Autodesk Inventor part; units mm, degrees
(part 3 of 3)
sketch "Sketch8" plane through (390.9, -150.3, 0) normal (0, 0, 1) x (0, 1, 0)
  line L0 (44.94, -15.18) -> (44.94, 14.82) projected
  line L1 (44.94, 14.82) -> (54.94, 14.82) projected
  line L2 (54.94, 14.82) -> (54.94, -15.18) projected
  line L3 (54.94, -15.18) -> (44.94, -15.18) projected
  line L4 (-55.06, -15.18) -> (-55.06, 14.82) projected
  line L5 (-55.06, 14.82) -> (-45.06, 14.82) projected
  line L6 (-45.06, 14.82) -> (-45.06, -15.18) projected
  line L7 (-45.06, -15.18) -> (-55.06, -15.18) projected
  circle A0 centre (56.765, -50.18) radius 1.7 projected
  circle A1 centre (56.765, 49.82) radius 1.7 projected
  circle A2 centre (-56.885, -50.18) radius 1.7 projected
  circle A3 centre (-56.885, 49.82) radius 1.7 projected
  line L8 (56.765, 74.82) -> (56.765, 86.645) projected
  line L9 (56.765, 86.645) -> (54.94, 86.645) projected
  line L10 (54.94, 86.645) -> (54.94, 89.82) projected
  line L11 (54.94, 89.82) -> (44.94, 89.82) projected
  line L12 (44.94, 89.82) -> (44.94, 86.645) projected
  line L13 (44.94, 86.645) -> (34.94, 86.645) projected
  line L14 (34.94, 86.645) -> (34.94, 89.82) projected
  line L15 (34.94, 89.82) -> (24.94, 89.82) projected
  line L16 (24.94, 89.82) -> (24.94, 86.645) projected
  line L17 (24.94, 86.645) -> (14.94, 86.645) projected
  line L18 (14.94, 86.645) -> (14.94, 89.82) projected
  line L19 (14.94, 89.82) -> (4.94, 89.82) projected
  line L20 (4.94, 89.82) -> (4.94, 86.645) projected
  line L21 (4.94, 86.645) -> (-5.06, 86.645) projected
  line L22 (-5.06, 86.645) -> (-5.06, 89.82) projected
  line L23 (-5.06, 89.82) -> (-15.06, 89.82) projected
  line L24 (-15.06, 89.82) -> (-15.06, 86.645) projected
  line L25 (-15.06, 86.645) -> (-25.06, 86.645) projected
  line L26 (-25.06, 86.645) -> (-25.06, 89.82) projected
  line L27 (-25.06, 89.82) -> (-35.06, 89.82) projected
  line L28 (-35.06, 89.82) -> (-35.06, 86.645) projected
  line L29 (-35.06, 86.645) -> (-45.06, 86.645) projected
  line L30 (-45.06, 86.645) -> (-45.06, 89.82) projected
  line L31 (-45.06, 89.82) -> (-55.06, 89.82) projected
  line L32 (-55.06, 89.82) -> (-55.06, 86.645) projected
  line L33 (-55.06, 86.645) -> (-56.885, 86.645) projected
  line L34 (-56.885, 86.645) -> (-56.885, 74.82) projected
  line L35 (-56.885, 74.82) -> (-60.06, 74.82) projected
  line L36 (-60.06, 74.82) -> (-60.06, 64.82) projected
  line L37 (-60.06, 64.82) -> (-56.885, 64.82) projected
  line L38 (-56.885, 64.82) -> (-56.885, 54.82) projected
  line L39 (-56.885, 54.82) -> (-60.06, 54.82) projected
  line L40 (-60.06, 54.82) -> (-60.06, 44.82) projected
  line L41 (-60.06, 44.82) -> (-56.885, 44.82) projected
  line L42 (-56.885, 44.82) -> (-56.885, 34.82) projected
  line L43 (-56.885, 34.82) -> (-60.06, 34.82) projected
  line L44 (-60.06, 34.82) -> (-60.06, 24.82) projected
  line L45 (-60.06, 24.82) -> (-56.885, 24.82) projected
  line L46 (-56.885, 24.82) -> (-56.885, 14.82) projected
  line L47 (-56.885, 14.82) -> (-60.06, 14.82) projected
  line L48 (-60.06, 14.82) -> (-60.06, 4.82) projected
  line L49 (-60.06, 4.82) -> (-56.885, 4.82) projected
  line L50 (-56.885, 4.82) -> (-56.885, -5.18) projected
  line L51 (-56.885, -5.18) -> (-60.06, -5.18) projected
  line L52 (-60.06, -5.18) -> (-60.06, -15.18) projected
  line L53 (-60.06, -15.18) -> (-56.885, -15.18) projected
  line L54 (-56.885, -15.18) -> (-56.885, -25.18) projected
  line L55 (-56.885, -25.18) -> (-60.06, -25.18) projected
  line L56 (-60.06, -25.18) -> (-60.06, -35.18) projected
  line L57 (-60.06, -35.18) -> (-56.885, -35.18) projected
  line L58 (-56.885, -35.18) -> (-56.885, -45.18) projected
  line L59 (-56.885, -45.18) -> (-60.06, -45.18) projected
  line L60 (-60.06, -45.18) -> (-60.06, -55.18) projected
  line L61 (-60.06, -55.18) -> (-56.885, -55.18) projected
  line L62 (-56.885, -55.18) -> (-56.885, -65.18) projected
  line L63 (-56.885, -65.18) -> (-60.06, -65.18) projected
  line L64 (-60.06, -65.18) -> (-60.06, -75.18) projected
  line L65 (-60.06, -75.18) -> (-56.885, -75.18) projected
  line L66 (-56.885, -75.18) -> (-56.885, -87.005) projected
  line L67 (-56.885, -87.005) -> (-55.06, -87.005) projected
  line L68 (-55.06, -87.005) -> (-55.06, -90.18) projected
  line L69 (-55.06, -90.18) -> (-45.06, -90.18) projected
  line L70 (-45.06, -90.18) -> (-45.06, -87.005) projected
  line L71 (-45.06, -87.005) -> (-35.06, -87.005) projected
  line L72 (-35.06, -87.005) -> (-35.06, -90.18) projected
  line L73 (-35.06, -90.18) -> (-25.06, -90.18) projected
  line L74 (-25.06, -90.18) -> (-25.06, -87.005) projected
  line L75 (-25.06, -87.005) -> (-15.06, -87.005) projected
  line L76 (-15.06, -87.005) -> (-15.06, -90.18) projected
  line L77 (-15.06, -90.18) -> (-5.06, -90.18) projected
  line L78 (-5.06, -90.18) -> (-5.06, -87.005) projected
  line L79 (-5.06, -87.005) -> (4.94, -87.005) projected
  line L80 (4.94, -87.005) -> (4.94, -90.18) projected
  line L81 (4.94, -90.18) -> (14.94, -90.18) projected
  line L82 (14.94, -90.18) -> (14.94, -87.005) projected
  line L83 (14.94, -87.005) -> (24.94, -87.005) projected
  line L84 (24.94, -87.005) -> (24.94, -90.18) projected
  line L85 (24.94, -90.18) -> (34.94, -90.18) projected
  line L86 (34.94, -90.18) -> (34.94, -87.005) projected
  line L87 (34.94, -87.005) -> (44.94, -87.005) projected
  line L88 (44.94, -87.005) -> (44.94, -90.18) projected
  line L89 (44.94, -90.18) -> (54.94, -90.18) projected
  line L90 (54.94, -90.18) -> (54.94, -87.005) projected
  line L91 (54.94, -87.005) -> (56.765, -87.005) projected
  line L92 (56.765, -87.005) -> (56.765, -75.18) projected
  line L93 (56.765, -75.18) -> (59.94, -75.18) projected
  line L94 (59.94, -75.18) -> (59.94, -65.18) projected
  line L95 (59.94, -65.18) -> (56.765, -65.18) projected
  line L96 (56.765, -65.18) -> (56.765, -55.18) projected
  line L97 (56.765, -55.18) -> (59.94, -55.18) projected
  line L98 (59.94, -55.18) -> (59.94, -45.18) projected
  line L99 (59.94, -45.18) -> (56.765, -45.18) projected
  line L100 (56.765, -45.18) -> (56.765, -35.18) projected
  line L101 (56.765, -35.18) -> (59.94, -35.18) projected
  line L102 (59.94, -35.18) -> (59.94, -25.18) projected
  line L103 (59.94, -25.18) -> (56.765, -25.18) projected
  line L104 (56.765, -25.18) -> (56.765, -15.18) projected
  line L105 (56.765, -15.18) -> (59.94, -15.18) projected
  line L106 (59.94, -15.18) -> (59.94, -5.18) projected
  line L107 (59.94, -5.18) -> (56.765, -5.18) projected
  line L108 (56.765, -5.18) -> (56.765, 4.82) projected
  line L109 (56.765, 4.82) -> (59.94, 4.82) projected
  line L110 (59.94, 4.82) -> (59.94, 14.82) projected
  line L111 (59.94, 14.82) -> (56.765, 14.82) projected
  line L112 (56.765, 14.82) -> (56.765, 24.82) projected
  line L113 (56.765, 24.82) -> (59.94, 24.82) projected
  line L114 (59.94, 24.82) -> (59.94, 34.82) projected
  line L115 (59.94, 34.82) -> (56.765, 34.82) projected
  line L116 (56.765, 34.82) -> (56.765, 44.82) projected
  line L117 (56.765, 44.82) -> (59.94, 44.82) projected
  line L118 (59.94, 44.82) -> (59.94, 54.82) projected
  line L119 (59.94, 54.82) -> (56.765, 54.82) projected
  line L120 (56.765, 54.82) -> (56.765, 64.82) projected
  line L121 (56.765, 64.82) -> (59.94, 64.82) projected
  line L122 (59.94, 64.82) -> (59.94, 74.82) projected
  line L123 (59.94, 74.82) -> (56.765, 74.82) projected
  line L124 (24.82, -87.125) -> (15.06, -87.125)
  line L125 (15.06, -87.125) -> (15.06, -90.3)
  line L126 (15.06, -90.3) -> (4.82, -90.3)
  line L127 (4.82, -90.3) -> (4.82, -87.125)
  line L128 (4.82, -87.125) -> (-4.94, -87.125)
  line L129 (-4.94, -87.125) -> (-4.94, -90.3)
  line L130 (-4.94, -90.3) -> (-15.18, -90.3)
  line L131 (-15.18, -90.3) -> (-15.18, -87.125)
  line L132 (-15.18, -87.125) -> (-24.94, -87.125)
  line L133 (-24.94, -87.125) -> (-24.94, -90.3)
  line L134 (-24.94, -90.3) -> (-35.18, -90.3)
  line L135 (-35.18, -90.3) -> (-35.18, -87.125)
  line L136 (-35.18, -87.125) -> (-44.94, -87.125)
  line L137 (-44.94, -87.125) -> (-44.94, -90.3)
  line L138 (-44.94, -90.3) -> (-55.18, -90.3)
  line L139 (-55.18, -90.3) -> (-55.18, -87.125)
  line L140 (-55.18, -87.125) -> (-57.005, -87.125)
  line L141 (-57.005, -87.125) -> (-57.005, -75.3)
  line L142 (-57.005, -75.3) -> (-60.18, -75.3)
  line L143 (-60.18, -75.3) -> (-60.18, -65.06)
  line L144 (-60.18, -65.06) -> (-57.005, -65.06)
  line L145 (-57.005, -65.06) -> (-57.005, -55.3)
  line L146 (-57.005, -55.3) -> (-60.18, -55.3)
  line L147 (-60.18, -55.3) -> (-60.18, -45.06)
  line L148 (-60.18, -45.06) -> (-57.005, -45.06)
  line L149 (-57.005, -45.06) -> (-57.005, -35.3)
  line L150 (-57.005, -35.3) -> (-60.18, -35.3)
  line L151 (-60.18, -35.3) -> (-60.18, -25.06)
  line L152 (-60.18, -25.06) -> (-57.005, -25.06)
  line L153 (-57.005, -25.06) -> (-57.005, -15.3)
  line L154 (-57.005, -15.3) -> (-60.18, -15.3)
  line L155 (-60.18, -15.3) -> (-60.18, -5.06)
  line L156 (-60.18, -5.06) -> (-57.005, -5.06)
  line L157 (-57.005, -5.06) -> (-57.005, 4.7)
  line L158 (-57.005, 4.7) -> (-60.18, 4.7)
  line L159 (-60.18, 4.7) -> (-60.18, 14.94)
  line L160 (-60.18, 14.94) -> (-57.005, 14.94)
  line L161 (-57.005, 14.94) -> (-57.005, 24.7)
  line L162 (-57.005, 24.7) -> (-60.18, 24.7)
  line L163 (-60.18, 24.7) -> (-60.18, 34.94)
  line L164 (-60.18, 34.94) -> (-57.005, 34.94)
  line L165 (-57.005, 34.94) -> (-57.005, 44.7)
  line L166 (-57.005, 44.7) -> (-60.18, 44.7)
  line L167 (-60.18, 44.7) -> (-60.18, 54.94)
  line L168 (-60.18, 54.94) -> (-57.005, 54.94)
  line L169 (-57.005, 54.94) -> (-57.005, 64.7)
  line L170 (-57.005, 64.7) -> (-60.18, 64.7)
  line L171 (-60.18, 64.7) -> (-60.18, 74.94)
  line L172 (-60.18, 74.94) -> (-57.005, 74.94)
  line L173 (-57.005, 74.94) -> (-57.005, 86.765)
  line L174 (-57.005, 86.765) -> (-55.18, 86.765)
  line L175 (-55.18, 86.765) -> (-55.18, 89.94)
  line L176 (-55.18, 89.94) -> (-44.94, 89.94)
  line L177 (-44.94, 89.94) -> (-44.94, 86.765)
  line L178 (-44.94, 86.765) -> (-35.18, 86.765)
  line L179 (-35.18, 86.765) -> (-35.18, 89.94)
  line L180 (-35.18, 89.94) -> (-24.94, 89.94)
  line L181 (-24.94, 89.94) -> (-24.94, 86.765)
  line L182 (-24.94, 86.765) -> (-15.18, 86.765)
  line L183 (-15.18, 86.765) -> (-15.18, 89.94)
  line L184 (-15.18, 89.94) -> (-4.94, 89.94)
  line L185 (-4.94, 89.94) -> (-4.94, 86.765)
  line L186 (-4.94, 86.765) -> (4.82, 86.765)
  line L187 (4.82, 86.765) -> (4.82, 89.94)
  line L188 (4.82, 89.94) -> (15.06, 89.94)
  line L189 (15.06, 89.94) -> (15.06, 86.765)
  line L190 (15.06, 86.765) -> (24.82, 86.765)
  line L191 (24.82, 86.765) -> (24.82, 89.94)
  line L192 (24.82, 89.94) -> (35.06, 89.94)
  line L193 (35.06, 89.94) -> (35.06, 86.765)
  line L194 (35.06, 86.765) -> (44.82, 86.765)
  line L195 (44.82, 86.765) -> (44.82, 89.94)
  line L196 (44.82, 89.94) -> (55.06, 89.94)
  line L197 (55.06, 89.94) -> (55.06, 86.765)
  line L198 (55.06, 86.765) -> (56.885, 86.765)
  line L199 (56.885, 86.765) -> (56.885, 74.94)
  line L200 (56.885, 74.94) -> (60.06, 74.94)
  line L201 (60.06, 74.94) -> (60.06, 64.7)
  line L202 (60.06, 64.7) -> (56.885, 64.7)
  line L203 (56.885, 64.7) -> (56.885, 54.94)
  line L204 (56.885, 54.94) -> (60.06, 54.94)
  line L205 (60.06, 54.94) -> (60.06, 44.7)
  line L206 (60.06, 44.7) -> (56.885, 44.7)
  line L207 (56.885, 44.7) -> (56.885, 34.94)
  line L208 (56.885, 34.94) -> (60.06, 34.94)
  line L209 (60.06, 34.94) -> (60.06, 24.7)
  line L210 (60.06, 24.7) -> (56.885, 24.7)
  line L211 (56.885, 24.7) -> (56.885, 14.94)
  line L212 (56.885, 14.94) -> (60.06, 14.94)
  line L213 (60.06, 14.94) -> (60.06, 4.7)
  line L214 (60.06, 4.7) -> (56.885, 4.7)
  line L215 (56.885, 4.7) -> (56.885, -5.06)
  line L216 (56.885, -5.06) -> (60.06, -5.06)
  line L217 (60.06, -5.06) -> (60.06, -15.3)
  line L218 (60.06, -15.3) -> (56.885, -15.3)
  line L219 (56.885, -15.3) -> (56.885, -25.06)
  line L220 (56.885, -25.06) -> (60.06, -25.06)
  line L221 (60.06, -25.06) -> (60.06, -35.3)
  line L222 (60.06, -35.3) -> (56.885, -35.3)
  line L223 (56.885, -35.3) -> (56.885, -45.06)
  line L224 (56.885, -45.06) -> (60.06, -45.06)
  line L225 (60.06, -45.06) -> (60.06, -55.3)
  line L226 (60.06, -55.3) -> (56.885, -55.3)
  line L227 (56.885, -55.3) -> (56.885, -65.06)
  line L228 (56.885, -65.06) -> (60.06, -65.06)
  line L229 (60.06, -65.06) -> (60.06, -75.3)
  line L230 (60.06, -75.3) -> (56.885, -75.3)
  line L231 (56.885, -75.3) -> (56.885, -87.125)
  line L232 (56.885, -87.125) -> (55.06, -87.125)
  line L233 (55.06, -87.125) -> (55.06, -90.3)
  line L234 (55.06, -90.3) -> (44.82, -90.3)
  line L235 (44.82, -90.3) -> (44.82, -87.125)
  line L236 (44.82, -87.125) -> (35.06, -87.125)
  line L237 (35.06, -87.125) -> (35.06, -90.3)
  line L238 (35.06, -90.3) -> (24.82, -90.3)
  line L239 (24.82, -90.3) -> (24.82, -87.125)
  circle A4 centre (56.765, -50.18) radius 1.58
  line L240 (45.06, -15.06) -> (45.06, 14.7)
  line L241 (45.06, 14.7) -> (54.82, 14.7)
  line L242 (54.82, 14.7) -> (54.82, -15.06)
  line L243 (54.82, -15.06) -> (45.06, -15.06)
  line L244 (-45.18, -15.06) -> (-45.18, 14.7)
  line L245 (-45.18, 14.7) -> (-54.94, 14.7)
  line L246 (-54.94, 14.7) -> (-54.94, -15.06)
  line L247 (-54.94, -15.06) -> (-45.18, -15.06)
  circle A5 centre (-56.885, 49.82) radius 1.58
  circle A6 centre (-56.885, -50.18) radius 1.58
  circle A7 centre (56.765, 49.82) radius 1.58
  point P0 (150.3, 390.9)
  dimension "d50" = 0.12
  dimension "d51" = 0.12
  dimension "d52" = 0.12
  dimension "d53" = 0.12
  dimension "d54" = 0.12
  dimension "d55" = 0.12
  dimension "d56" = 0.12
  constraints: 248 end point, 4 centre point, 121 other
  measures "d50" distance between parallel lines of L83 L124
  measures "d51" radial gap between concentric circles of A0 A4
  measures "d52" distance between parallel lines of L3 L243
  measures "d53" distance between parallel lines of L6 L244
  measures "d54" radial gap between concentric circles of A3 A5
  measures "d55" radial gap between concentric circles of A2 A6
  measures "d56" radial gap between concentric circles of A1 A7
extrude "Extrusion8" add sketch "Sketch8" along normal blind 3.175 contours L0 L1 L2 L3 | L4 L5 L6 L7 | A0 | A1 | A2 | A3 | L123 L122 L121 L120 L119 L118 L117 L116 L115 L114 L113 L112 L111 L110 L109 L108 L107 L106 L105 L104 L103 L102 L101 L100 L99 L98 L97 L96 L95 L94 L93 L92 L91 L90 L89 L88 L87 L86 L85 L84 L83 L82 L81 L80 L79 L78 L77 L76 L75 L74 L73 L72 L71 L70 L69 L68 L67 L66 L65 L64 L63 L62 L61 L60 L59 L58 L57 L56 L55 L54 L53 L52 L51 L50 L49 L48 L47 L46 L45 L44 L43 L42 L41 L40 L39 L38 L37 L36 L35 L34 L33 L32 L31 L30 L29 L28 L27 L26 L25 L24 L23 L22 L21 L20 L19 L18 L17 L16 L15 L14 L13 L12 L11 L10 L9 L8
ref_plane "Work Plane8" through (481.2, 0, 0) normal (0, 0, 1) x (1, 0, 0)
sketch "Sketch9" plane through (481.2, 0, 0) normal (0, 0, 1) x (1, 0, 0)
  line L0 (44.055, -13.335) -> (40.245, -13.335) projected
  line L1 (40.245, -13.335) -> (40.245, -1.905) projected
  line L2 (40.245, -1.905) -> (44.055, -1.905) projected
  line L3 (44.055, -1.905) -> (44.055, -13.335) projected
  circle A0 centre (38.34, -15.24) radius 1.078 projected
  circle A1 centre (45.96, 0) radius 1.078 projected
  circle A2 centre (45.96, -15.24) radius 1.078 projected
  circle A3 centre (38.34, 0) radius 1.078 projected
  line L4 (55.065, -48.5) -> (57.065, -48.5) projected
  line L5 (57.065, -48.5) -> (57.065, -45) projected
  line L6 (57.065, -45) -> (60.24, -45) projected
  line L7 (60.24, -45) -> (60.24, -35) projected
  line L8 (60.24, -35) -> (57.065, -35) projected
  line L9 (57.065, -35) -> (57.065, -25) projected
  line L10 (57.065, -25) -> (60.24, -25) projected
  line L11 (60.24, -25) -> (60.24, -15) projected
  line L12 (60.24, -15) -> (57.065, -15) projected
  line L13 (57.065, -15) -> (57.065, -5) projected
  line L14 (57.065, -5) -> (60.24, -5) projected
  line L15 (60.24, -5) -> (60.24, 5) projected
  line L16 (60.24, 5) -> (57.065, 5) projected
  line L17 (57.065, 5) -> (57.065, 15) projected
  line L18 (57.065, 15) -> (60.24, 15) projected
  line L19 (60.24, 15) -> (60.24, 25) projected
  line L20 (60.24, 25) -> (57.065, 25) projected
  line L21 (57.065, 25) -> (57.065, 35) projected
  line L22 (57.065, 35) -> (60.24, 35) projected
  line L23 (60.24, 35) -> (60.24, 45) projected
  line L24 (60.24, 45) -> (57.065, 45) projected
  line L25 (57.065, 45) -> (57.065, 48.5) projected
  line L26 (57.065, 48.5) -> (55.065, 48.5) projected
  line L27 (55.065, 48.5) -> (55.065, 47.25) projected
  line L28 (55.065, 47.25) -> (52.565, 47.25) projected
  line L29 (52.565, 47.25) -> (52.565, 48.5) projected
  line L30 (52.565, 48.5) -> (46.24, 48.5) projected
  line L31 (46.24, 48.5) -> (46.24, 51.5) projected
  line L32 (46.24, 51.5) -> (52.565, 51.5) projected
  line L33 (52.565, 51.5) -> (52.565, 52.75) projected
  line L34 (52.565, 52.75) -> (55.065, 52.75) projected
  line L35 (55.065, 52.75) -> (55.065, 51.5) projected
  line L36 (55.065, 51.5) -> (57.065, 51.5) projected
  line L37 (57.065, 51.5) -> (57.065, 55) projected
  line L38 (57.065, 55) -> (60.24, 55) projected
  line L39 (60.24, 55) -> (60.24, 65) projected
  line L40 (60.24, 65) -> (57.065, 65) projected
  line L41 (57.065, 65) -> (57.065, 75) projected
  line L42 (57.065, 75) -> (60.24, 75) projected
  line L43 (60.24, 75) -> (60.24, 86.825) projected
  line L44 (55.24, 86.825) -> (60.24, 86.825) projected
  line L45 (55.24, 90) -> (55.24, 86.825) projected
  line L46 (45.24, 90) -> (55.24, 90) projected
  line L47 (45.24, 86.825) -> (45.24, 90) projected
  line L48 (45.24, 86.825) -> (35.24, 86.825) projected
  line L49 (35.24, 90) -> (35.24, 86.825) projected
  line L50 (25.24, 90) -> (35.24, 90) projected
  line L51 (25.24, 86.825) -> (25.24, 90) projected
  line L52 (25.24, 86.825) -> (15.24, 86.825) projected
  line L53 (15.24, 90) -> (15.24, 86.825) projected
  line L54 (5.24, 90) -> (15.24, 90) projected
  line L55 (5.24, 86.825) -> (5.24, 90) projected
  line L56 (5.24, 86.825) -> (-4.76, 86.825) projected
  line L57 (-4.76, 90) -> (-4.76, 86.825) projected
  line L58 (-14.76, 90) -> (-4.76, 90) projected
  line L59 (-14.76, 86.825) -> (-14.76, 90) projected
  line L60 (-14.76, 86.825) -> (-24.76, 86.825) projected
  line L61 (-24.76, 90) -> (-24.76, 86.825) projected
  line L62 (-34.76, 90) -> (-24.76, 90) projected
  line L63 (-34.76, 86.825) -> (-34.76, 90) projected
  line L64 (-34.76, 86.825) -> (-44.76, 86.825) projected
  line L65 (-44.76, 90) -> (-44.76, 86.825) projected
  line L66 (-54.76, 90) -> (-44.76, 90) projected
  line L67 (-54.76, 86.825) -> (-54.76, 90) projected
  line L68 (-54.76, 86.825) -> (-59.76, 86.825) projected
  line L69 (-59.76, 75) -> (-59.76, 86.825) projected
  line L70 (-56.585, 75) -> (-59.76, 75) projected
  line L71 (-56.585, 75) -> (-56.585, 65) projected
  line L72 (-59.76, 65) -> (-56.585, 65) projected
  line L73 (-59.76, 55) -> (-59.76, 65) projected
  line L74 (-56.585, 55) -> (-59.76, 55) projected
  line L75 (-56.585, 55) -> (-56.585, 45) projected
  line L76 (-59.76, 45) -> (-56.585, 45) projected
  line L77 (-59.76, 35) -> (-59.76, 45) projected
  line L78 (-56.585, 35) -> (-59.76, 35) projected
  line L79 (-56.585, 35) -> (-56.585, 25) projected
  line L80 (-59.76, 25) -> (-56.585, 25) projected
  line L81 (-59.76, 15) -> (-59.76, 25) projected
  line L82 (-56.585, 15) -> (-59.76, 15) projected
  line L83 (-56.585, 15) -> (-56.585, 5) projected
  line L84 (-59.76, 5) -> (-56.585, 5) projected
  line L85 (-59.76, -5) -> (-59.76, 5) projected
  line L86 (-56.585, -5) -> (-59.76, -5) projected
  line L87 (-56.585, -5) -> (-56.585, -15) projected
  line L88 (-59.76, -15) -> (-56.585, -15) projected
  line L89 (-59.76, -25) -> (-59.76, -15) projected
  line L90 (-56.585, -25) -> (-59.76, -25) projected
  line L91 (-56.585, -25) -> (-56.585, -35) projected
  line L92 (-59.76, -35) -> (-56.585, -35) projected
  line L93 (-59.76, -45) -> (-59.76, -35) projected
  line L94 (-56.585, -45) -> (-59.76, -45) projected
  line L95 (-56.585, -45) -> (-56.585, -55) projected
  line L96 (-59.76, -55) -> (-56.585, -55) projected
  line L97 (-59.76, -65) -> (-59.76, -55) projected
  line L98 (-56.585, -65) -> (-59.76, -65) projected
  line L99 (-56.585, -65) -> (-56.585, -75) projected
  line L100 (-59.76, -75) -> (-56.585, -75) projected
  line L101 (-59.76, -75) -> (-59.76, -86.825) projected
  line L102 (-59.76, -86.825) -> (-54.76, -86.825) projected
  line L103 (-54.76, -86.825) -> (-54.76, -90) projected
  line L104 (-54.76, -90) -> (-44.76, -90) projected
  line L105 (-44.76, -90) -> (-44.76, -86.825) projected
  line L106 (-44.76, -86.825) -> (-34.76, -86.825) projected
  line L107 (-34.76, -86.825) -> (-34.76, -90) projected
  line L108 (-34.76, -90) -> (-24.76, -90) projected
  line L109 (-24.76, -90) -> (-24.76, -86.825) projected
  line L110 (-24.76, -86.825) -> (-14.76, -86.825) projected
  line L111 (-14.76, -86.825) -> (-14.76, -90) projected
  line L112 (-14.76, -90) -> (-4.76, -90) projected
  line L113 (-4.76, -90) -> (-4.76, -86.825) projected
  line L114 (-4.76, -86.825) -> (5.24, -86.825) projected
  line L115 (5.24, -86.825) -> (5.24, -90) projected
  line L116 (5.24, -90) -> (15.24, -90) projected
  line L117 (15.24, -90) -> (15.24, -86.825) projected
  line L118 (15.24, -86.825) -> (25.24, -86.825) projected
  line L119 (25.24, -86.825) -> (25.24, -90) projected
  line L120 (25.24, -90) -> (35.24, -90) projected
  line L121 (35.24, -90) -> (35.24, -86.825) projected
  line L122 (35.24, -86.825) -> (45.24, -86.825) projected
  line L123 (45.24, -86.825) -> (45.24, -90) projected
  line L124 (45.24, -90) -> (55.24, -90) projected
  line L125 (55.24, -90) -> (55.24, -86.825) projected
  line L126 (55.24, -86.825) -> (60.24, -86.825) projected
  line L127 (60.24, -86.825) -> (60.24, -75) projected
  line L128 (60.24, -75) -> (57.065, -75) projected
  line L129 (57.065, -75) -> (57.065, -65) projected
  line L130 (57.065, -65) -> (60.24, -65) projected
  line L131 (60.24, -65) -> (60.24, -55) projected
  line L132 (60.24, -55) -> (57.065, -55) projected
  line L133 (57.065, -55) -> (57.065, -51.5) projected
  line L134 (57.065, -51.5) -> (55.065, -51.5) projected
  line L135 (55.065, -51.5) -> (55.065, -52.75) projected
  line L136 (55.065, -52.75) -> (52.565, -52.75) projected
  line L137 (52.565, -52.75) -> (52.565, -51.5) projected
  line L138 (52.565, -51.5) -> (46.24, -51.5) projected
  line L139 (46.24, -51.5) -> (46.24, -48.5) projected
  line L140 (46.24, -48.5) -> (52.565, -48.5) projected
  line L141 (52.565, -48.5) -> (52.565, -47.25) projected
  line L142 (52.565, -47.25) -> (55.065, -47.25) projected
  line L143 (55.065, -47.25) -> (55.065, -48.5) projected
  circle A4 centre (23.2372, -27.4451) radius 3 projected
  circle A5 centre (-22.7572, 54) radius 3 projected
  circle A6 centre (23.2372, 27.4451) radius 3 projected
  circle A7 centre (-22.7572, -54) radius 3 projected
  circle A8 centre (-14.76, 8.175) radius 11 projected
  line L144 (-44.64, 90.12) -> (-44.64, 86.945)
  line L145 (-44.64, 86.945) -> (-34.88, 86.945)
  line L146 (-34.88, 86.945) -> (-34.88, 90.12)
  line L147 (-34.88, 90.12) -> (-24.64, 90.12)
  line L148 (-24.64, 90.12) -> (-24.64, 86.945)
  line L149 (-24.64, 86.945) -> (-14.88, 86.945)
  line L150 (-14.88, 86.945) -> (-14.88, 90.12)
  line L151 (-14.88, 90.12) -> (-4.64, 90.12)
  line L152 (-4.64, 90.12) -> (-4.64, 86.945)
  line L153 (-4.64, 86.945) -> (5.12, 86.945)
  line L154 (5.12, 86.945) -> (5.12, 90.12)
  line L155 (5.12, 90.12) -> (15.36, 90.12)
  line L156 (15.36, 90.12) -> (15.36, 86.945)
  line L157 (15.36, 86.945) -> (25.12, 86.945)
  line L158 (25.12, 86.945) -> (25.12, 90.12)
  line L159 (25.12, 90.12) -> (35.36, 90.12)
  line L160 (35.36, 90.12) -> (35.36, 86.945)
  line L161 (35.36, 86.945) -> (45.12, 86.945)
  line L162 (45.12, 86.945) -> (45.12, 90.12)
  line L163 (45.12, 90.12) -> (55.36, 90.12)
  line L164 (55.36, 90.12) -> (55.36, 86.945)
  line L165 (55.36, 86.945) -> (60.36, 86.945)
  line L166 (60.36, 86.945) -> (60.36, 74.88)
  line L167 (60.36, 74.88) -> (57.185, 74.88)
  line L168 (57.185, 74.88) -> (57.185, 65.12)
  line L169 (57.185, 65.12) -> (60.36, 65.12)
  line L170 (60.36, 65.12) -> (60.36, 54.88)
  line L171 (60.36, 54.88) -> (57.185, 54.88)
  line L172 (57.185, 54.88) -> (57.185, 51.38)
  line L173 (57.185, 51.38) -> (54.945, 51.38)
  line L174 (54.945, 51.38) -> (54.945, 52.63)
  line L175 (54.945, 52.63) -> (52.685, 52.63)
  line L176 (52.685, 52.63) -> (52.685, 51.38)
  line L177 (52.685, 51.38) -> (46.36, 51.38)
  line L178 (46.36, 51.38) -> (46.36, 48.62)
  line L179 (46.36, 48.62) -> (52.685, 48.62)
  line L180 (52.685, 48.62) -> (52.685, 47.37)
  line L181 (52.685, 47.37) -> (54.945, 47.37)
  line L182 (54.945, 47.37) -> (54.945, 48.62)
  line L183 (54.945, 48.62) -> (57.185, 48.62)
  line L184 (57.185, 48.62) -> (57.185, 45.12)
  line L185 (57.185, 45.12) -> (60.36, 45.12)
  line L186 (60.36, 45.12) -> (60.36, 34.88)
  line L187 (60.36, 34.88) -> (57.185, 34.88)
  line L188 (57.185, 34.88) -> (57.185, 25.12)
  line L189 (57.185, 25.12) -> (60.36, 25.12)
  line L190 (60.36, 25.12) -> (60.36, 14.88)
  line L191 (60.36, 14.88) -> (57.185, 14.88)
  line L192 (57.185, 14.88) -> (57.185, 5.12)
  line L193 (57.185, 5.12) -> (60.36, 5.12)
  line L194 (60.36, 5.12) -> (60.36, -5.12)
  line L195 (60.36, -5.12) -> (57.185, -5.12)
  line L196 (57.185, -5.12) -> (57.185, -14.88)
  line L197 (57.185, -14.88) -> (60.36, -14.88)
  line L198 (60.36, -14.88) -> (60.36, -25.12)
  line L199 (60.36, -25.12) -> (57.185, -25.12)
  line L200 (57.185, -25.12) -> (57.185, -34.88)
  line L201 (57.185, -34.88) -> (60.36, -34.88)
  line L202 (60.36, -34.88) -> (60.36, -45.12)
  line L203 (60.36, -45.12) -> (57.185, -45.12)
  line L204 (57.185, -45.12) -> (57.185, -48.62)
  line L205 (57.185, -48.62) -> (54.945, -48.62)
  line L206 (54.945, -48.62) -> (54.945, -47.37)
  line L207 (54.945, -47.37) -> (52.685, -47.37)
  line L208 (52.685, -47.37) -> (52.685, -48.62)
  line L209 (52.685, -48.62) -> (46.36, -48.62)
  line L210 (46.36, -48.62) -> (46.36, -51.38)
  line L211 (46.36, -51.38) -> (52.685, -51.38)
  line L212 (52.685, -51.38) -> (52.685, -52.63)
  line L213 (52.685, -52.63) -> (54.945, -52.63)
  line L214 (54.945, -52.63) -> (54.945, -51.38)
  line L215 (54.945, -51.38) -> (57.185, -51.38)
  line L216 (57.185, -51.38) -> (57.185, -54.88)
  line L217 (57.185, -54.88) -> (60.36, -54.88)
  line L218 (60.36, -54.88) -> (60.36, -65.12)
  line L219 (60.36, -65.12) -> (57.185, -65.12)
  line L220 (57.185, -65.12) -> (57.185, -74.88)
  line L221 (57.185, -74.88) -> (60.36, -74.88)
  line L222 (60.36, -74.88) -> (60.36, -86.945)
  line L223 (60.36, -86.945) -> (55.36, -86.945)
  line L224 (55.36, -86.945) -> (55.36, -90.12)
  line L225 (55.36, -90.12) -> (45.12, -90.12)
  line L226 (45.12, -90.12) -> (45.12, -86.945)
  line L227 (45.12, -86.945) -> (35.36, -86.945)
  line L228 (35.36, -86.945) -> (35.36, -90.12)
  line L229 (35.36, -90.12) -> (25.12, -90.12)
  line L230 (25.12, -90.12) -> (25.12, -86.945)
  line L231 (25.12, -86.945) -> (15.36, -86.945)
  line L232 (15.36, -86.945) -> (15.36, -90.12)
  line L233 (15.36, -90.12) -> (5.12, -90.12)
  line L234 (5.12, -90.12) -> (5.12, -86.945)
  line L235 (5.12, -86.945) -> (-4.64, -86.945)
  line L236 (-4.64, -86.945) -> (-4.64, -90.12)
  line L237 (-4.64, -90.12) -> (-14.88, -90.12)
  line L238 (-14.88, -90.12) -> (-14.88, -86.945)
  line L239 (-14.88, -86.945) -> (-24.64, -86.945)
  line L240 (-24.64, -86.945) -> (-24.64, -90.12)
  line L241 (-24.64, -90.12) -> (-34.88, -90.12)
  line L242 (-34.88, -90.12) -> (-34.88, -86.945)
  line L243 (-34.88, -86.945) -> (-44.64, -86.945)
  line L244 (-44.64, -86.945) -> (-44.64, -90.12)
  line L245 (-44.64, -90.12) -> (-54.88, -90.12)
  line L246 (-54.88, -90.12) -> (-54.88, -86.945)
  line L247 (-54.88, -86.945) -> (-59.88, -86.945)
  line L248 (-59.88, -86.945) -> (-59.88, -74.88)
  line L249 (-59.88, -74.88) -> (-56.705, -74.88)
  line L250 (-56.705, -74.88) -> (-56.705, -65.12)
  line L251 (-56.705, -65.12) -> (-59.88, -65.12)
  line L252 (-59.88, -65.12) -> (-59.88, -54.88)
  line L253 (-59.88, -54.88) -> (-56.705, -54.88)
  line L254 (-56.705, -54.88) -> (-56.705, -45.12)
  line L255 (-56.705, -45.12) -> (-59.88, -45.12)
  line L256 (-59.88, -45.12) -> (-59.88, -34.88)
  line L257 (-59.88, -34.88) -> (-56.705, -34.88)
  line L258 (-56.705, -34.88) -> (-56.705, -25.12)
  line L259 (-56.705, -25.12) -> (-59.88, -25.12)
  line L260 (-59.88, -25.12) -> (-59.88, -14.88)
  line L261 (-59.88, -14.88) -> (-56.705, -14.88)
  line L262 (-56.705, -14.88) -> (-56.705, -5.12)
  line L263 (-56.705, -5.12) -> (-59.88, -5.12)
  line L264 (-59.88, -5.12) -> (-59.88, 5.12)
  line L265 (-59.88, 5.12) -> (-56.705, 5.12)
  line L266 (-56.705, 5.12) -> (-56.705, 14.88)
  line L267 (-56.705, 14.88) -> (-59.88, 14.88)
  line L268 (-59.88, 14.88) -> (-59.88, 25.12)
  line L269 (-59.88, 25.12) -> (-56.705, 25.12)
  line L270 (-56.705, 25.12) -> (-56.705, 34.88)
  line L271 (-56.705, 34.88) -> (-59.88, 34.88)
  line L272 (-59.88, 34.88) -> (-59.88, 45.12)
  line L273 (-59.88, 45.12) -> (-56.705, 45.12)
  line L274 (-56.705, 45.12) -> (-56.705, 54.88)
  line L275 (-56.705, 54.88) -> (-59.88, 54.88)
  line L276 (-59.88, 54.88) -> (-59.88, 65.12)
  line L277 (-59.88, 65.12) -> (-56.705, 65.12)
  line L278 (-56.705, 65.12) -> (-56.705, 74.88)
  line L279 (-56.705, 74.88) -> (-59.88, 74.88)
  line L280 (-59.88, 74.88) -> (-59.88, 86.945)
  line L281 (-59.88, 86.945) -> (-54.88, 86.945)
  line L282 (-54.88, 86.945) -> (-54.88, 90.12)
  line L283 (-54.88, 90.12) -> (-44.64, 90.12)
  circle A9 centre (-22.7572, 54) radius 2.88
  circle A10 centre (-14.76, 8.175) radius 10.88
  circle A11 centre (-22.7572, -54) radius 2.88
  circle A12 centre (23.2372, -27.4451) radius 2.88
  circle A13 centre (23.2372, 27.4451) radius 2.88
  line L284 (40.365, -2.025) -> (40.365, -13.215)
  line L285 (40.365, -13.215) -> (43.935, -13.215)
  line L286 (43.935, -13.215) -> (43.935, -2.025)
  line L287 (43.935, -2.025) -> (40.365, -2.025)
  circle A14 centre (45.96, 0) radius 0.958
  circle A15 centre (38.34, 0) radius 0.958
  circle A16 centre (38.34, -15.24) radius 0.958
  circle A17 centre (45.96, -15.24) radius 0.958
  point P0 (-481.2, 0)
  dimension "d59" = 0.12
  dimension "d60" = 0.12
  dimension "d61" = 0.12
  dimension "d62" = 0.12
  dimension "d63" = 0.12
  dimension "d64" = 0.12
  dimension "d65" = 0.12
  dimension "d66" = 0.12
  dimension "d67" = 0.12
  dimension "d68" = 0.12
  dimension "d69" = 0.12
  constraints: 288 end point, 9 centre point, 142 other
  measures "d59" distance between parallel lines of L66 L283
  measures "d60" radial gap between concentric circles of A5 A9
  measures "d61" radial gap between concentric circles of A8 A10
  measures "d62" radial gap between concentric circles of A7 A11
  measures "d63" radial gap between concentric circles of A4 A12
  measures "d64" radial gap between concentric circles of A6 A13
  measures "d65" distance between parallel lines of L1 L284
  measures "d66" radial gap between concentric circles of A1 A14
  measures "d67" radial gap between concentric circles of A3 A15
  measures "d68" radial gap between concentric circles of A0 A16
  measures "d69" radial gap between concentric circles of A2 A17
extrude "Extrusion9" add sketch "Sketch9" along normal blind 3.175 contours L0 L1 L2 L3 | A0 | A1 | A2 | A3 | L143 L142 L141 L140 L139 L138 L137 L136 L135 L134 L133 L132 L131 L130 L129 L128 L127 L126 L125 L124 L123 L122 L121 L120 L119 L118 L117 L116 L115 L114 L113 L112 L111 L110 L109 L108 L107 L106 L105 L104 L103 L102 L101 L100 L99 L98 L97 L96 L95 L94 L93 L92 L91 L90 L89 L88 L87 L86 L85 L84 L83 L82 L81 L80 L79 L78 L77 L76 L75 L74 L73 L72 L71 L70 L69 L68 L67 L66 L65 L64 L63 L62 L61 L60 L59 L58 L57 L56 L55 L54 L53 L52 L51 L50 L49 L48 L47 L46 L45 L44 L43 L42 L41 L40 L39 L38 L37 L36 L35 L34 L33 L32 L31 L30 L29 L28 L27 L26 L25 L24 L23 L22 L21 L20 L19 L18 L17 L16 L15 L14 L13 L12 L11 L10 L9 L8 L7 L6 L5 L4 | A4 | A5 | A6 | A7 | A8
equation "\"d0\" = laserKerf"
equation "\"d1\" = laserKerf"
equation "\"d2\" = laserKerf"
equation "\"d3\" = laserKerf"
equation "\"d4\" = laserKerf"
equation "\"d5\" = laserKerf"
equation "\"d6\" = laserKerf"
equation "\"d7\" = laserKerf"
equation "\"d8\" = laserKerf"
equation "\"d9\" = laserKerf"
equation "\"d10\" = laserKerf"
equation "\"d11\" = laserKerf"
equation "\"d12\" = laserKerf"
equation "\"d13\" = materialThickness"
equation "\"d15\" = laserKerf"
equation "\"d16\" = laserKerf"
equation "\"d17\" = laserKerf"
equation "\"d18\" = laserKerf"
equation "\"d19\" = laserKerf"
equation "\"d20\" = laserKerf"
equation "\"d21\" = laserKerf"
equation "\"d22\" = materialThickness"
equation "\"d24\" = laserKerf"
equation "\"d25\" = laserKerf"
equation "\"d26\" = materialThickness"
equation "\"d28\" = laserKerf"
equation "\"d29\" = laserKerf"
equation "\"d30\" = laserKerf"
equation "\"d31\" = laserKerf"
equation "\"d32\" = laserKerf"
equation "\"d33\" = laserKerf"
equation "\"d34\" = laserKerf"
equation "\"d35\" = laserKerf"
equation "\"d36\" = laserKerf"
equation "\"d37\" = laserKerf"
equation "\"d38\" = laserKerf"
equation "\"d39\" = materialThickness"
equation "\"d41\" = laserKerf"
equation "\"d42\" = materialThickness"
equation "\"d44\" = laserKerf"
equation "\"d45\" = materialThickness"
equation "\"d47\" = laserKerf"
equation "\"d48\" = materialThickness"
equation "\"d50\" = laserKerf"
equation "\"d51\" = laserKerf"
equation "\"d52\" = laserKerf"
equation "\"d53\" = laserKerf"
equation "\"d54\" = laserKerf"
equation "\"d55\" = laserKerf"
equation "\"d56\" = laserKerf"
equation "\"d57\" = materialThickness"
equation "\"d59\" = laserKerf"
equation "\"d60\" = laserKerf"
equation "\"d61\" = laserKerf"
equation "\"d62\" = laserKerf"
equation "\"d63\" = laserKerf"
equation "\"d64\" = laserKerf"
equation "\"d65\" = laserKerf"
equation "\"d66\" = laserKerf"
equation "\"d67\" = laserKerf"
equation "\"d68\" = laserKerf"
equation "\"d69\" = laserKerf"
equation "\"d70\" = materialThickness"
equation "\"materialThickness\" = 3.175"
equation "\"laserKerf\" = 0.12"
equation "\"cardPinDiameter\" = 3"
equation "\"centeralShaftDiameter\" = 8"
equation "\"cardWidth\" = 85.6"
equation "\"cardHeight\" = 53.98"
equation "\"cardThickness\" = 0.76"
equation "\"cardFillet\" = 2.88"
equation "\"cardClearence\" = 0.5"
equation "\"bearingOd\" = 22"
equation "\"bearingWidth\" = 8"
equation "\"axleHeight\" = 95"
equation "\"nutTrapClearence\" = 2"
equation "\"nutTrapwidth\" = 5.5"
equation "\"nutTrapDepth\" = 2.5"
equation "\"magnetDiameter\" = 6"
equation "\"magnetLength\" = 3"
equation "\"magnetProtusion\" = 0.25"
equation "\"spoolThickness\" = 5.588"
body "Solid1"
